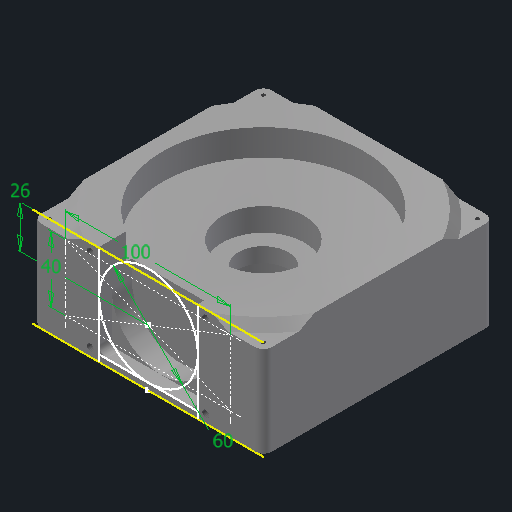
# Autodesk Inventor part: soporte de rodamientos
Saved by Autodesk Inventor 2022 (Build 260153000, 153)
## iProperties
Created: 2021-09-08
Part Number: soporte de rodamientos
Material: Aluminum 6061
Document SubType Name: Modeling
Designer: Andres
Density: 2.7 g/cm^3
Appearance: Steel
Author: Andres
Autodesk Inventor part; units mm, degrees
ref_plane "YZ Plane" through (0, 0, 0) normal (1, 0, 0) x (0, 1, 0)
ref_plane "XZ Plane" through (0, 0, 0) normal (0, 1, 0) x (-1, 0, 0)
ref_plane "XY Plane" through (0, 0, 0) normal (0, 0, 1) x (1, 0, 0)
sketch "Sketch8" plane through (0, 0, 0) normal (0, 1, 0) x (-1, 0, 0)
  circle A0 centre (0, 0) radius 15
  line L0 (70, 130) -> (-70, 130)
  line L1 (-70, 130) -> (-70, -70)
  line L2 (-70, -70) -> (70, -70)
  line L3 (70, -70) -> (70, 130)
  line L4 (70, 70) -> (-70, 70)
  point P0 (0, -70)
  dimension "d71" = 200
  dimension "d72" = 30
  dimension "d73" = 140
  dimension "d74" = 70
  dimension "d152" = 70
  constraints: 10 end point, 2 parallel, 2 perpendicular, 2 point on line, 1 centre point, 1 coincident, 1 horizontal, 1 midpoint, 1 vertical alignment
  measures "d71" distance of L2.end L0.start
  measures "d72" diameter of A0
  measures "d73" distance between parallel lines of L3 L1
  measures "d74" distance from line of point (0, 0) L2
  measures "d152" distance from line of point (0, 0) L4
extrude "Extrusion10" add sketch "Sketch8" along normal blind 60 contours L3 L2 L1 L4
ref_plane "Work Plane6" through (-21.2011, 20.6833, -21.2011) normal (0, -1, 0) x (0.7306278, 0, -0.6827759)
sketch "Sketch9" plane through (0, 60, 0) normal (0, 1, 0) x (1, 0, 0)
  circle A0 centre (0, 0) radius 25
  circle A1 centre (0, 0) radius 15 projected
  dimension "d81" = 50
  constraints: 1 centre point, 1 coincident
  measures "d81" diameter of A0
extrude "Extrusion11" cut sketch "Sketch9" against normal blind 30
sketch "Sketch15" plane through (-70, 0, 70) normal (0, 0, 1) x (1, 0, 0)
  line L0 (20, 54) -> (120, 54) construction
  line L1 (120, 54) -> (120, 14) construction
  line L2 (120, 14) -> (20, 14) construction
  line L3 (20, 14) -> (20, 54) construction
  line L4 (20, 54) -> (120, 14) construction
  line L5 (120, 54) -> (20, 14) construction
  line L6 (0, 0) -> (140, 0) projected
  circle A0 centre (70, 34) radius 30
  line L7 (0, 60) -> (140, 60) projected
  line L8 (40, 34) -> (40, 60)
  line L9 (100, 34) -> (100, 60)
  line L10 (40, 34) -> (40, 0)
  line L11 (100, 34) -> (100, 0)
  line L12 (40, 4) -> (100, 4)
  point P0 (70, 0)
  point P1 (70, 34)
  point P2 (70, 34)
  point P3 (70, 0)
  point P4 (84.9666, 60)
  point P5 (55.0334, 60)
  point P6 (70, 4)
  dimension "d140" = 100
  dimension "d141" = 40
  dimension "d143" = 60
  dimension "d151" = 26
  constraints: 22 end point, 5 coincident, 5 midpoint, 4 perpendicular, 4 point on line, 3 tangent, 2 parallel, 2 point on circle, 2 vertical, 1 centre point, 1 horizontal, 1 vertical alignment, 3 other
  measures "d140" distance of L0.start L0.end
  measures "d141" distance of L2.end L0.start
  measures "d143" diameter of A0
extrude "Extrusion19" cut sketch "Sketch15" against normal blind 20 contours L8 L7 A0 | A0 L7 | A0 L7 L9 | A0 L7
ref_plane "Work Plane5" through (-60.7764, 61.8111, -60.7764) normal (0, -1, 0) x (0.7306278, 0, -0.6827759)
ref_plane "Work Plane7" through (-60.7764, 56.8111, -60.7764) normal (0, -1, 0) x (0.7306278, 0, -0.6827759)
sketch "Sketch17" plane through (-70, 0, 70) normal (0, 0, 1) x (1, 0, 0)
  point P0 (70, 0)
sketch "Sketch20" plane through (0, 60, 0) normal (0, 1, 0) x (1, 0, 0)
  circle A0 centre (0, 0) radius 61
  dimension "d158" = 122
  constraints: 1 centre point, 1 coincident
  measures "d158" diameter of A0
extrude "Extrusion23" cut sketch "Sketch20" against normal blind 16
extrude "Extrusion24" cut sketch "Sketch15" against normal blind 8 contours L10 A0 L12 | L12 A0 L11 | A0 L7 picked at (68.9573, 61.2788)
fillet "Fillet5" radius 5 2 edges at (-30, 4, 66) (30, 4, 66)
sketch "Sketch21" plane through (-70, 0, 70) normal (0, 0, 1) x (1, 0, 0)
  circle A0 centre (35, 5) radius 2.65 projected
  circle A1 centre (35, 55) radius 2.65 projected
  circle A2 centre (105, 55) radius 2.65 projected
  circle A3 centre (105, 5) radius 2.65 projected
  point P0 (70, 0)
hole "Hole4" at (-35, 55, 70) at (-35, 5, 70) at (35, 5, 70) at (35, 55, 70) direction (0, 0, -1) diameter 4.134 depth 14.2 tip angle 118 thread size "M5x0.8" class "6H" standard "ISO Metric profile"
sketch "Sketch23" plane through (0, 60, 0) normal (0, 1, 0) x (1, 0, 0)
  circle A0 centre (0, 0) radius 85
  arc A1 (30, -53.1131) -> (-30, -53.1131) centre (0, 0) ccw projected
  line L0 (30, -53.1131) -> (30, -70) projected
  line L1 (30, -70) -> (70, -70) projected
  line L2 (70, -70) -> (70, 70) projected
  line L3 (70, 70) -> (-70, 70) projected
  line L4 (-70, 70) -> (-70, -70) projected
  line L5 (-70, -70) -> (-30, -70) projected
  line L6 (-30, -70) -> (-30, -53.1131) projected
  point P0 (70, -48.2183)
  point P1 (48.2183, -70)
  point P2 (48.2183, 70)
  point P3 (70, 48.2183)
  point P4 (-70, 48.2183)
  point P5 (-48.2183, 70)
  point P6 (-48.2183, -70)
  point P7 (-70, -48.2183)
  dimension "d182" = 170
  constraints: 1 centre point, 1 coincident
  measures "d182" diameter of A0
extrude "Extrusion25" cut sketch "Sketch23" against normal blind 5 contours A0 L3 L2 | L2 L1 A0 | A0 L4 L3 | L5 L4 A0
chamfer "Chamfer6" distance 5 angle 45 4 edges at (60.1041, 60, 60.1041) (60.1041, 60, -60.1041) (-60.1041, 60, -60.1041) (-60.1041, 60, 60.1041)
sketch "Sketch22" plane through (0, 55, 0) normal (0, 1, 0) x (1, 0, 0)
  arc A0 (30, -53.1131) -> (-30, -53.1131) centre (0, 0) ccw projected
  line L0 (30, -53.1131) -> (30, -70) projected
  line L1 (30, -70) -> (38.7298, -70) projected
  line L2 (70, -38.7298) -> (70, 38.7298) projected
  line L3 (38.7298, 70) -> (-38.7298, 70) projected
  line L4 (-70, 38.7298) -> (-70, -38.7298) projected
  line L5 (-38.7298, -70) -> (-30, -70) projected
  line L6 (-30, -70) -> (-30, -53.1131) projected
  line L7 (65, -65) -> (-65, -65) construction
  line L8 (-65, -65) -> (-65, 65) construction
  line L9 (-65, 65) -> (65, 65) construction
  line L10 (65, 65) -> (65, -65) construction
  line L11 (65, -65) -> (-65, 65) construction
  line L12 (-65, -65) -> (65, 65) construction
  arc A1 (-70, -38.7298) -> (-38.7298, -70) centre (0, 0) ccw projected
  arc A2 (38.7298, -70) -> (70, -38.7298) centre (0, 0) ccw projected
  arc A3 (70, 38.7298) -> (38.7298, 70) centre (0, 0) ccw projected
  arc A4 (-38.7298, 70) -> (-70, 38.7298) centre (0, 0) ccw projected
  dimension "d172" = 130
  dimension "d173" = 130
  constraints: 12 end point, 2 midpoint, 2 parallel, 1 horizontal, 1 perpendicular
  measures "d172" distance of L8.end L9.end
  measures "d173" distance of L7.end L8.end
hole "Hole5" at (-65, 55, 65) at (65, 55, 65) at (65, 55, -65) at (-65, 55, -65) direction (0, -1, 0) diameter 2.459 depth 8.8 tip angle 118 thread size "M3x0.5" class "6H" standard "ISO Metric profile"
fillet "Fillet6" radius 5 4 edges at (70, 27.5, 70) (70, 27.5, -70) (-70, 27.5, -70) (-70, 27.5, 70)
sketch "Sketch24" plane through (0, 0, 0) normal (0, -1, 0) x (1, 0, 0)
  circle A0 centre (0, 0) radius 26
  dimension "d188" = 52
  constraints: 1 centre point, 1 coincident
  measures "d188" diameter of A0
extrude "Extrusion26" cut sketch "Sketch24" against normal blind 21
sketch "Sketch25" plane through (0, 0, 0) normal (0, -1, 0) x (1, 0, 0)
  circle A0 centre (0, 0) radius 40 projected
  circle A1 centre (0, 0) radius 26 projected
  point P0 (0, 0)
extrude "Extrusion27" cut sketch "Sketch25" against normal blind 8
sketch "Sketch26" plane through (0, 21, 0) normal (0, -1, 0) x (1, 0, 0)
  circle A0 centre (0, 0) radius 26 projected
  circle A1 centre (0, 0) radius 24
  dimension "d193" = 2
  constraints: 1 centre point
  measures "d193" radial gap between concentric circles of A0 A1
extrude "Extrusion28" add sketch "Sketch26" along normal blind 0.5
body "Solid3"
